holderbase (Autodesk Fusion 360 design; units mm, degrees)
Autodesk Fusion 360 part; units mm, degrees
sketch "Sketch1" plane through (0, 0, 0) normal (0, 1, 0) x (1, 0, 0)
  line L0 (0, 0) -> (35, -80)
  line L1 (35, -80) -> (65, -80)
  line L2 (65, -80) -> (100, 0)
  line L3 (100, 0) -> (0, 0)
  circle A0 centre (50, -50) radius 7.5
  circle A1 centre (50, -50) radius 3
  line L4 (100, 0) -> (0, 0)
  line L5 (0, 0) -> (0, 5)
  line L6 (0, 5) -> (100, 5)
  line L7 (100, 5) -> (100, 0)
  dimension "d1" = 100
  dimension "d2" = 30
  dimension "d4" = 80
  dimension "d5" = 35
  dimension "d6" = 50
  dimension "d7" = 15
  dimension "d8" = 15
  dimension "d13" = 6
  dimension "d15" = 5
  constraint horizontal L1
  constraint parallel L1 L3
  constraint coincident L0.start L3.end
  constraint concentric A0 A1
  constraint horizontal L4
  constraint vertical L5
  constraint horizontal L6
  constraint vertical L7
  measures "d1" distance of L0.start L2.end
  measures "d2" distance of L0.end L1.end
  measures "d4" distance of L1 L3
  measures "d5" horizontal distance of L0.start L0.end
  measures "d6" vertical distance of L0.start A0.centre
  measures "d7" diameter of A0
  measures "d8" horizontal distance of L1.end A0.centre
  measures "d13" diameter of A1
  measures "d15" distance of L0.start L5.end
extrude "Extrude3" add sketch "Sketch1" along normal blind 44 contours L3 L4 L5 L6 L7
